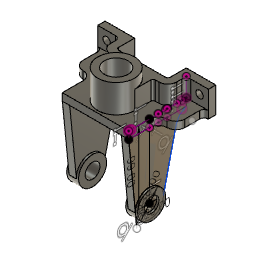
Surprise Checkpoint Q2 v1 (Autodesk Fusion 360 design; units mm, degrees)
Autodesk Fusion 360 part; units mm, degrees
sketch "Sketch1" plane through (0, 0, 0) normal (0, 0, 1) x (1, 0, 0)
  line L0 (27.2139, 50) -> (94.2139, 50)
  line L1 (27.2139, 50) -> (27.2139, 75)
  line L2 (97.2139, 53) -> (97.2139, 75)
  line L3 (27.2139, 75) -> (-12.7861, 75)
  line L4 (97.2139, 75) -> (137.2139, 75)
  line L5 (27.2139, 75) -> (97.2139, 75) construction
  line L6 (62.2139, 75) -> (62.2139, 15) construction
  circle A0 centre (62.2139, 15) radius 25
  circle A1 centre (62.2139, 15) radius 16
  line L7 (-12.7861, 75) -> (-12.7861, 65)
  line L8 (-12.7861, 65) -> (15, 65)
  line L9 (17.2139, 55.9638) -> (17.2139, 40)
  line L10 (90.2139, 40) -> (99.6926, 40)
  line L11 (107.2139, 53.2502) -> (107.2139, 59)
  line L12 (113.2139, 65) -> (143.3083, 65)
  line L13 (15, 65) -> (17.2139, 65)
  line L14 (17.2139, 55.9638) -> (17.2139, 65)
  line L15 (99.6926, 40) -> (95.2139, 40)
  line L16 (107.2139, 52) -> (107.2139, 53.2502)
  line L17 (87.2139, 15) -> (87.2139, 37)
  line L18 (37.2139, 15) -> (37.2139, 40)
  arc A2 (90.2139, 40) -> (87.2139, 37) centre (90.2139, 37) ccw
  arc A3 (95.2139, 40) -> (107.2139, 52) centre (95.2139, 52) ccw
  arc A4 (113.2139, 65) -> (107.2139, 59) centre (113.2139, 59) ccw
  arc A5 (94.2139, 50) -> (97.2139, 53) centre (94.2139, 53) ccw
  line L19 (62.2139, 75) -> (62.2139, -24.3763) construction
  line L20 (62.2139, 75) -> (62.2139, -24.3763) construction
  line L21 (34.2139, 40) -> (24.7352, 40)
  line L22 (11.2139, 65) -> (-18.8805, 65)
  line L23 (-18.8805, 65) -> (-18.8805, 75)
  arc A6 (17.2139, 52) -> (29.2139, 40) centre (29.2139, 52) ccw
  line L24 (24.7352, 40) -> (29.2139, 40)
  line L25 (17.2139, 53.2502) -> (17.2139, 59)
  line L26 (97.2139, 75) -> (27.2139, 75) construction
  arc A7 (17.2139, 59) -> (11.2139, 65) centre (11.2139, 59) ccw
  line L27 (-18.8805, 75) -> (-12.7861, 75)
  line L28 (17.2139, 52) -> (17.2139, 53.2502)
  circle A8 centre (62.2139, 15) radius 16
  line L29 (37.2139, 15) -> (37.2139, 37)
  line L30 (97.2139, 50) -> (30.2139, 50)
  arc A9 (27.2139, 53) -> (30.2139, 50) centre (30.2139, 53) ccw
  line L31 (27.2139, 53) -> (27.2139, 75)
  line L32 (27.2139, 75) -> (-12.7861, 75)
  arc A10 (37.2139, 37) -> (34.2139, 40) centre (34.2139, 37) ccw
  circle A11 centre (62.2139, 15) radius 25
  line L33 (137.2139, 75) -> (137.2139, 65)
  point P0 (97.2139, 50)
  point P1 (27.2139, 50)
  dimension "d6" = 70
  dimension "d7" = 25
  dimension "d8" = 25
  dimension "d9" = 40
  dimension "d10" = 40
  dimension "d11" = 60
  dimension "d12" = 50
  dimension "d13" = 32
  dimension "d14" = 10
  dimension "d15" = 10
  dimension "d16" = 10
  dimension "d17" = 10
  dimension "d18" = 10
  dimension "d19" = 3
  dimension "d20" = 12
  dimension "d21" = 6
  dimension "d22" = 3
  constraint horizontal L0
  constraint perpendicular L0 L1
  constraint perpendicular L0 L2
  constraint perpendicular L1 L3
  constraint perpendicular L2 L4
  constraint midpoint L5 L6.start
  constraint perpendicular L5 L6
  constraint coincident L6.end A0.centre
  constraint concentric A0 A1
  constraint perpendicular L3 L7
  constraint perpendicular L7 L8
  constraint vertical L9
  constraint perpendicular L6 L10
  constraint parallel L6 L11
  constraint perpendicular L11 L12
  constraint perpendicular L9 L13
  constraint perpendicular L13 L14
  constraint perpendicular L11 L15
  constraint perpendicular L15 L16
  constraint coincident A0 L17.start
  constraint perpendicular L10 L17
  constraint tangent A0 L17
  constraint coincident A0 L18.start
  constraint coincident L10 L18.end
  constraint perpendicular L10 L18
  constraint tangent A0 L18
  constraint coincident L9.end L10
  constraint tangent L17 A2
  constraint tangent L10 A2
  constraint tangent L16 A3
  constraint tangent L15 A3
  constraint tangent L12 A4
  constraint tangent L11 A4
  constraint coincident P0 L2
  constraint tangent L2 A5
  constraint tangent L0 A5
  constraint parallel L6 L19
  constraint symmetric L0.start L6 P0
  constraint symmetric P0 L6 P1
  constraint symmetric L1.end L6 L2.end
  constraint symmetric L2.end L6 L1.end
  constraint symmetric L4.end L6 L3.end
  constraint symmetric L19.start L6 L20.start
  constraint symmetric L6 A0 A11
  constraint symmetric L6 A1 A8
  constraint symmetric L6 L10.end L21.end
  constraint symmetric L6 L11.start L25.start
  constraint symmetric L6 L12.end L22.end
  constraint symmetric L6 L17.start L18.start
  constraint symmetric L6 L17.end L29.end
  constraint symmetric L6 L10.start L21.start
  constraint symmetric L6 A2 A10
  constraint symmetric L6 L16.start A6.start
  constraint symmetric L6 L15.end A6.end
  constraint symmetric L6 A3 A6
  constraint symmetric L6 L12.start L22.start
  constraint symmetric L6 L11.end L25.end
  constraint symmetric L6 A4 A7
  constraint symmetric L6 L2.start A9.start
  constraint symmetric L6 L0.end L30.end
  constraint symmetric L6 A5 A9
  constraint symmetric L6 L19.end L20.end
  constraint coincident L12 L33.end
  constraint perpendicular L12 L33
  measures "d6" distance of L0.start P0
  measures "d7" distance of L0.start L1.end
  measures "d8" distance of P0 L2.end
  measures "d9" distance of L1.end L3.end
  measures "d10" distance of L2.end L4.end
  measures "d11" distance of L6.start L6.end
  measures "d12" diameter of A0
  measures "d13" diameter of A1
  measures "d14" distance of L3.end L7.end
  measures "d15" distance of L0 L10
  measures "d16" distance of L1 L14
  measures "d17" distance of L2 L11
  measures "d18" distance of L4 L12
  measures "d19" radius of A2
  measures "d20" radius of A3
  measures "d21" radius of A4
  measures "d22" radius of A5
extrude "Extrude1" add sketch "Sketch1" along normal blind 38 contours A0 A11 makes body 1
extrude "Extrude2" add sketch "Sketch1" along normal blind 25 contours L0 L1 L2 L3 L4 A0 L7 L8 L9 L10 L11 L12 L13 L14 L16 L17 L18 A2 A3 A4 A5 L21 L22 A6 L25 L28 L29 L30 L31 L32 A10 A11 L33 bodies 1
fillet "Fillet1" radius 3 1 edges at (27.2139, 50, 12.5) on bodies 1
sketch "Sketch2" plane through (0, 0, 0) normal (0, 0, -1) x (1, 0, 0)
  circle A0 centre (62.2139, -15) radius 16
  arc A1 (87.2139, -15) -> (37.2139, -15) centre (62.2139, -15) ccw
  line L0 (37.2139, -15) -> (37.2139, -37)
  arc A2 (34.2139, -40) -> (37.2139, -37) centre (34.2139, -37) ccw
  line L1 (34.2139, -40) -> (29.2139, -40)
  arc A3 (29.2139, -40) -> (17.2139, -52) centre (29.2139, -52) ccw
  line L2 (17.2139, -52) -> (17.2139, -65)
  line L3 (17.2139, -65) -> (-12.7861, -65)
  line L4 (-12.7861, -65) -> (-12.7861, -75)
  line L5 (-12.7861, -75) -> (27.2139, -75)
  line L6 (27.2139, -75) -> (27.2139, -53)
  arc A4 (30.2139, -50) -> (27.2139, -53) centre (30.2139, -53) ccw
  line L7 (30.2139, -50) -> (94.2139, -50)
  arc A5 (97.2139, -53) -> (94.2139, -50) centre (94.2139, -53) ccw
  line L8 (97.2139, -53) -> (97.2139, -75)
  line L9 (97.2139, -75) -> (137.2139, -75)
  line L10 (137.2139, -65) -> (113.2139, -65)
  arc A6 (107.2139, -59) -> (113.2139, -65) centre (113.2139, -59) ccw
  line L11 (107.2139, -59) -> (107.2139, -52)
  arc A7 (107.2139, -52) -> (95.2139, -40) centre (95.2139, -52) ccw
  line L12 (95.2139, -40) -> (90.2139, -40)
  arc A8 (87.2139, -37) -> (90.2139, -40) centre (90.2139, -37) ccw
  line L13 (87.2139, -37) -> (87.2139, -15)
  line L14 (-12.7861, -75) -> (-12.7861, -65)
  line L15 (27.2139, -75) -> (97.2139, -75)
  line L16 (62.2139, -75) -> (62.2139, 13)
  line L17 (62.2139, 13) -> (107.2139, 13)
  line L18 (62.2139, -15) -> (37.2139, -15)
  line L19 (62.2139, -15) -> (107.2139, -15)
  line L20 (107.2139, -15) -> (107.2139, 13)
  line L21 (107.2139, -15) -> (107.2139, -14.5244)
  line L22 (137.2139, -65) -> (129, -65)
  line L23 (131.2139, -65) -> (131.2139, -48)
  line L24 (107.2139, -14.5244) -> (113.2139, -14.5244)
  line L25 (113.2139, -14.5244) -> (119.2139, -14.5244)
  line L26 (107.2139, -15) -> (119.2139, -15)
  arc A9 (107.2139, -15) -> (119.2139, -27) centre (119.2139, -15) ccw
  line L27 (119.2139, -15) -> (107.2139, -15) construction
  line L28 (119.2139, -15) -> (119.2139, -27) construction
  line L29 (108.6237, -27) -> (129, -27)
  line L30 (119.2139, -27) -> (125.3083, -37.3372)
  line L31 (131.2139, -48) -> (131.2139, -39)
  line L32 (129, -27) -> (119.2139, -27)
  arc A10 (131.2139, -39) -> (119.2139, -27) centre (119.2139, -39) ccw
  arc A11 (131.2139, -59) -> (137.2139, -65) centre (137.2139, -59) ccw
  line L33 (62.2139, -89.3776) -> (62.2139, 44.3933)
  line L34 (137.2139, -75) -> (137.2139, -65)
  dimension "d28" = 88
  dimension "d30" = 45
  dimension "d41" = 12
  dimension "d42" = 6
  dimension "d43" = 6
  dimension "d44" = 12
  dimension "d45" = 90
  dimension "d48" = 12
  dimension "d50" = 12
  constraint coincident L4.end L5.start
  constraint coincident L3.end L4.start
  constraint coincident L5.end L6.start
  constraint coincident L8.end L9.start
  constraint midpoint L15 L16.start
  constraint perpendicular L7 L16
  constraint perpendicular L16 L17
  constraint coincident A0.centre A1.centre
  constraint perpendicular L13 L19
  constraint perpendicular L17 L20
  constraint perpendicular L19 L21
  constraint coincident L10.start L22.start
  constraint coincident L10 L22.end
  constraint tangent L22 A11
  constraint collinear L9.end L10.start A11.centre
  constraint coincident L10 L23.start
  constraint perpendicular L22 L23
  constraint tangent L23 A11
  constraint perpendicular L20 L24
  constraint perpendicular L21 L26
  constraint coincident L26.end A9.centre
  constraint parallel L23 L31
  constraint perpendicular L31 L32
  constraint tangent L32 A10
  constraint tangent L31 A10
  constraint coincident L23 A11.start
  constraint perpendicular L18 L33
  measures "d28" distance of L16.start L16.end
  measures "d30" distance of L16.end L17.end
  measures "d41" diameter of A11
  measures "d42" distance of L21.end L24.end
  measures "d43" distance of L24.end L25.end
  measures "d44" distance of L19.end L26.end
  measures "d45" angle of L27 L28
  measures "d48" distance of A9.end L30.end
  measures "d50" radius of A10
sketch "Sketch3" plane through (0, 0, 0) normal (0, 0, -1) x (1, 0, 0)
extrude "Extrude3" add sketch "Sketch2" along normal blind 10 separate body contours L10 A6 L11 A7 L12 A8 L13 L19 L22 L23 A9 L31 A10 | A1 L16 L17 L19 L20 L21 L33 makes body 2
extrude "Extrude4" add sketch "Sketch1" against normal blind 10 contours L0 L1 L2 L3 L4 A0 L7 L8 L9 L10 L11 L12 L13 L14 L16 L17 L18 A2 A3 A4 A5 L21 L22 A6 L25 L28 L29 L30 L31 L32 A10 A11 L33 bodies 1 2
ref_plane "WorkPlane1" through (62.2139, 64, 7.5) normal (-1, 0, 0) x (0, -1, 0)
mirror "Mirror1" about plane through (62.2139, 64, 7.5) normal (-1, 0, 0) of bodies 1 makes body 3
combine "Combine1" operation add target body 1 tool bodies 3
fillet "Fillet2" radius 6 1 edges at (-6.7861, 65, -5) on bodies 1
fillet "Fillet3" radius 6 1 edges at (131.2139, 65, -5) on bodies 1
ref_plane "WorkPlane2" through (107.2139, -13, 0) normal (-1, 0, 0) x (0, -1, 0)
sketch "Sketch4" plane through (107.2139, -13, 0) normal (-1, 0, 0) x (0, 1, 0)
  line L0 (28, 0) -> (28, 10)
  line L1 (28, 0) -> (0, 0)
  line L2 (40, 0) -> (28, 0)
  line L3 (40, 0) -> (40, 10)
  line L4 (28, 10) -> (40, 10)
  line L5 (28, 10) -> (0, 10)
  line L6 (72, 0) -> (52, 0)
  line L7 (72, 10) -> (52, 10)
  line L8 (52, 0) -> (40, 0)
  line L9 (52, 10) -> (40, 10)
  line L10 (28, 0) -> (28, 99)
  circle A0 centre (28, 99) radius 19
  circle A1 centre (28, 99) radius 10
  line L11 (0, 10) -> (10.9973, 119.9093)
  line L12 (0, 10) -> (78, 10)
  line L13 (47, 99) -> (64.0336, 25.8302)
  arc A2 (64.0336, 25.8302) -> (78, 10) centre (85.7068, 30.8756) ccw
  line L14 (78, 0) -> (78, -25)
  line L15 (78, -25) -> (78, 0)
  line L16 (53, 0) -> (50, 0)
  line L17 (50, 0) -> (28, 0)
  line L18 (3, 0) -> (28, 0)
  line L19 (28, 0) -> (50, 0)
  line L20 (53, 0) -> (50, 0)
  line L21 (53, 0) -> (65, 0)
  line L22 (65, 0) -> (72, 0)
  line L23 (72, 0) -> (78, 0)
  line L24 (72, 0) -> (78, 0)
  line L25 (72, 0) -> (52, 0)
  line L26 (40, 0) -> (52, 0)
  line L27 (28, 0) -> (40, 0)
  line L28 (28, 0) -> (0, 0)
  line L29 (0, 0) -> (28, 0)
  line L30 (40, 0) -> (28, 0)
  line L31 (52, 0) -> (40, 0)
  line L32 (52, 0) -> (72, 0)
  line L33 (72, 0) -> (78, 0)
  line L34 (78, 0) -> (72, 0)
  line L35 (72, 0) -> (65, 0)
  line L36 (53, 0) -> (65, 0)
  line L37 (78, 0) -> (78, 10)
  point P0 (78, 0)
  dimension "d58" = 99
  dimension "d59" = 38
  dimension "d61" = 20
  constraint coincident L0.start L1.start
  constraint perpendicular L1 L10
  constraint coincident L10.end A0.centre
  constraint concentric A0 A1
  constraint coincident L5.end L11.start
  constraint tangent A0 L11
  constraint perpendicular L10 L12
  constraint coincident A0 L13.start
  constraint tangent L13 A2
  constraint coincident P0 L14.start
  constraint coincident L12 A2.end
  constraint perpendicular L12 L37
  measures "d58" distance of L0.start L10.end
  measures "d59" diameter of A0
  measures "d61" diameter of A1
extrude "Extrude5" add sketch "Sketch4" along normal blind 10 separate body contours L4 L7 L9 L10 A0 L12 L13 A2 | L5 L10 A0 L11 L12 makes body 4
extrude "Extrude6" add sketch "Sketch4" along normal blind 13 and the other way blind 3 separate body contours A0 makes body 5
hole "Hole1" at (125.2139, 65, 13) direction (0, 1, 0) diameter 10 depth 10 tip angle 180 bodies 1
mirror "Mirror2" about plane through (62.2139, 64, 7.5) normal (-1, 0, 0) of bodies 4 5 makes body 6 at (30.2139, 15, -83.0354) makes body 7 at (17.2139, 3.926, -33.5772)
hole "Hole2" at (-0.7861, 65, 13) direction (0, 1, 0) diameter 10 depth 10 tip angle 180 bodies 1
